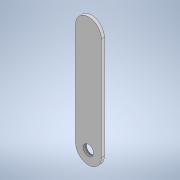
# Autodesk Inventor part: 零件1
Saved by Autodesk Inventor 2022 (Build 260153000, 153)
## iProperties
Created: 2023-04-19
Part Number: 零件1
Material: 一般
Document SubType Name: Modeling
Designer: JOU
Density: 1 g/cm^3
Appearance: 預設
Author: JOU
Autodesk Inventor part; units mm, degrees
ref_plane "YZ Plane" through (0, 0, 0) normal (1, 0, 0) x (0, 1, 0)
ref_plane "XZ Plane" through (0, 0, 0) normal (0, 1, 0) x (-1, 0, 0)
ref_plane "XY Plane" through (0, 0, 0) normal (0, 0, 1) x (1, 0, 0)
sketch "草圖1" plane through (0, 0, 0) normal (0, 0, 1) x (1, 0, 0)
  circle A0 centre (0, 0) radius 5
  line L0 (0, 0) -> (0, 100) construction
  line L1 (12.5, 0) -> (12.5, 100)
  line L2 (-12.5, 100) -> (-12.5, 0)
  arc A1 (-12.5, 0) -> (12.5, 0) centre (0, 0) ccw
  arc A2 (12.5, 100) -> (-12.5, 100) centre (0, 100) ccw
  point P0 (0, 50)
  dimension "d0" = 10
  dimension "d1" = 100
  dimension "d2" = 25
  constraints: 8 end point, 4 point on circle, 4 tangent, 3 centre point, 1 coincident, 1 midpoint, 1 parallel, 1 vertical
  measures "d0" diameter of A0
  measures "d1" distance of L0.start L0.end
  measures "d2" diameter of A2
extrude "擠出1" add sketch "草圖1" along normal blind 3
